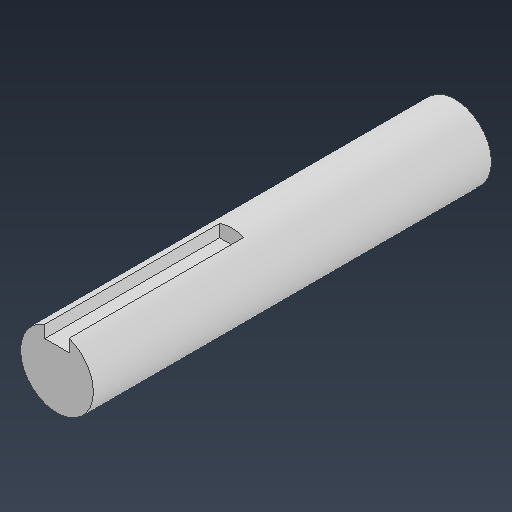
# Autodesk Inventor part: MCEN4000:P1
Saved by Autodesk Inventor 2021 (Build 250183000, 183)
## iProperties
Created: 2020-10-17
Part Number: MCEN4000:P1
Material: Generic
Document SubType Name: Modeling
Designer: Eugene Tang
Mass: 32.5311 g
Surface Area: 97.0063 cm^2
Volume: 32.5311 cm^3
Density: 1 g/cm^3
Appearance: Default
Description: Intermediate Gear Pin
GearPin_DIA: 15.000 mm
Bearing_WIDTH: 11.000 mm
Bearing_OD: 35.000 mm
IMKEY_D: 3.000 mm
Author: Eugene Tang
Autodesk Inventor part; units mm, degrees
ref_plane "YZ Plane" through (0, 0, 0) normal (1, 0, 0) x (0, 1, 0)
ref_plane "XZ Plane" through (0, 0, 0) normal (0, 1, 0) x (-1, 0, 0)
ref_plane "XY Plane" through (0, 0, 0) normal (0, 0, 1) x (1, 0, 0)
sketch "Sketch1" plane through (0, 0, 0) normal (0, 0, 1) x (1, 0, 0)
  circle A0 centre (0, 0) radius 47.888 construction
  circle A1 centre (-120, 0) radius 21.2836 construction
  line L0 (-120, 0) -> (0, 0) construction
  circle A2 centre (0, 0) radius 33
  circle A3 centre (-73.5661, -11.7112) radius 26.6044 construction
  dimension "d0" = 95.776
  dimension "d1" = 42.5671
  dimension "d4" = 120
  dimension "d16" = 66
  dimension "d17" = 53.2089
  constraints: 4 centre point, 2 coincident, 2 end point, 2 tangent, 1 horizontal
  measures "d0" diameter of A0
  measures "d1" diameter of A1
  measures "d4" distance of L0.start L0.end
  measures "d16" diameter of A2
  measures "d17" diameter of A3
sketch "Sketch2" plane through (0, 0, 0) normal (0, 0, 1) x (1, 0, 0)
  circle A0 centre (-120, 0) radius 7.5
  circle A1 centre (-120, 0) radius 21.2836 construction
  circle A2 centre (-73.5661, 11.7112) radius 26.6044 construction
  line L0 (-120, 0) -> (-100.9074, 0) construction
  line L1 (-120, 0) -> (-120, 23.2296) construction
  point P0 (0, 0)
  dimension "d5" = 15
  constraints: 4 end point, 1 centre point, 1 concentric, 1 horizontal, 1 vertical
  measures "d5" diameter of A0
extrude "Extrusion1" add sketch "Sketch2" along normal blind 65 and the other way blind 40
sketch "Sketch4" plane through (0, 0, 0) normal (0, 0, 1) x (1, 0, 0)
  circle A0 centre (-73.5661, -11.7112) radius 7.5
  circle A1 centre (-73.5661, -11.7112) radius 26.6044 construction
  line L0 (-73.5661, -11.7112) -> (-73.5661, 40.9362) construction
  line L1 (-73.5661, -11.7112) -> (-109.3594, -11.7112) construction
  point P0 (0, 0)
  dimension "d18" = 15
  constraints: 4 end point, 1 centre point, 1 concentric, 1 horizontal, 1 vertical
  measures "d18" diameter of A0
extrude "Extrusion3" add sketch "Sketch4" along normal blind 16 and the other way blind 66 separate body
sketch3d "3D Sketch1"
ref_plane "Work Plane1" through (-73.5661, -11.7112, 48.9351) normal (1, 0, 0) x (0, 0, -1)
sketch3d "3D Sketch2"
ref_plane "Work Plane2" through (-120, 0, 0) normal (1, 0, 0) x (0, 1, 0)
sketch "Sketch5" plane through (-73.5661, -11.7112, 16) normal (0, 0, 1) x (1, 0, 0)
  circle A0 centre (0, 0) radius 7.5 construction
  line L0 (0, 0) -> (0, 31.0502) construction
  line L1 (-14.5269, 7.5) -> (19.4754, 7.5) construction
  line L2 (-2.5, 9.5) -> (-2.5, 4.5)
  line L3 (-2.5, 4.5) -> (2.5, 4.5)
  line L4 (2.5, 4.5) -> (2.5, 9.5)
  line L5 (2.5, 9.5) -> (-2.5, 9.5)
  point P0 (73.5661, 11.7112)
  point P1 (2.5, 7.5)
  point P2 (0, 9.5)
  dimension "d23" = 5
  dimension "IMKEY_D" = 3
  constraints: 12 end point, 3 parallel, 3 perpendicular, 2 point on line, 1 midpoint, 1 tangent, 1 vertical
  measures "d23" distance of L3.end L4.end
  measures "IMKEY_D" distance between parallel lines of L1 L3
extrude "Extrusion4" cut sketch "Sketch5" against normal blind 36 bodies 2
equation "\"d0\" = d3"
equation "\"d1\" = d3_1"
equation "\"d16\" = Nut_OD"
equation "\"d17\" = d3_1_2"
equation "\"d5\" = Pin_DIA"
equation "\"d9\" = d1_1 + Hub_L"
equation "\"d18\" = GearPin_DIA"
equation "\"d23\" = IMKEY_W"
equation "\"IdleGearPin_L\" = 1"
equation "\"Bearing_WIDTH\" = 11"
equation "\"Pin_DIA\" = GearPin_DIA"
equation "\"TD\" = 0.45"
equation "\"Ball_DIA\" = 6"
equation "\"Screw_L\" = 292"
equation "\"Screw_DIA\" = 36"
equation "\"Nut_OD\" = 66"
equation "\"BPath_REVQ\" = 5.75"
equation "\"Tread_OFFSET\" = 8.075"
equation "\"SteeringColumn_DIA\" = 26"
equation "\"SteeringColumnChamfer_DEG\" = 20deg"
equation "\"Rack_L\" = 307.252"
equation "\"NutCapTread_L\" = 25"
equation "\"NutCapTread_THICKNESS\" = 5.365"
equation "\"SupportFlange_THICKNESS\" = 5"
equation "\"Bearing_OD\" = 35"
equation "\"GearKey_L\" = 32"
equation "\"d3\" = 95.776"
equation "\"d3_1\" = 42.567111"
equation "\"d3_1_2\" = 53.208889"
equation "\"d1_1\" = 30"
equation "\"Hub_L\" = 10"
equation "\"GearPin_DIA\" = 15"
equation "\"IMKEY_W\" = 5"
body "Solid1"
body "Solid2"
